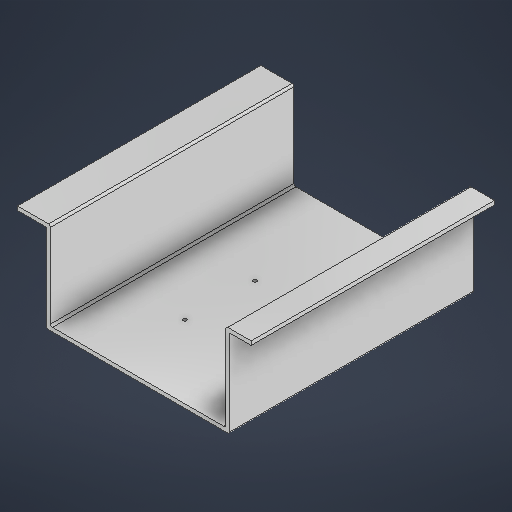
# Autodesk Inventor part: Lower joint housing
Saved by Autodesk Inventor 2026.3 (Build 303398000, 398)
## iProperties
Created: 2026-07-26
Part Number: Lower joint housing
Material: Generic
Document SubType Name: Sheet Metal
Designer: matot
Density: 1 g/cm^3
Sheet Metal Rule: Default_mm
Appearance: Default
Author: matot
Autodesk Inventor part; units mm, degrees
ref_plane "YZ Plane" through (0, 0, 0) normal (1, 0, 0) x (0, 1, 0)
ref_plane "XZ Plane" through (0, 0, 0) normal (0, 1, 0) x (-1, 0, 0)
ref_plane "XY Plane" through (0, 0, 0) normal (0, 0, 1) x (1, 0, 0)
sketch "Sketch1" plane through (0, 0, 0) normal (0, 0, 1) x (1, 0, 0)
  line L0 (98, 0) -> (98, -90)
  line L1 (98, -90) -> (-90, -90)
  line L2 (-90, -90) -> (-90, 0)
  line L3 (120, 4) -> (120, 0)
  line L4 (120, 0) -> (-120, 0)
  line L5 (-120, 0) -> (-120, 4)
  line L6 (-86, 4) -> (94, 4)
  line L7 (94, 4) -> (94, -86)
  line L8 (94, -86) -> (-86, -86)
  line L9 (-86, -86) -> (-86, 4)
  line L10 (-90, 0) -> (-86, 0)
  line L11 (94, 0) -> (98, 0)
  line L12 (-120, 4) -> (-86, 4)
  line L13 (94, 4) -> (120, 4)
  point P0 (0, 0)
  point P1 (0, -4)
  point P2 (120, 2)
  point P3 (98, 0)
  dimension "d0" = 188
  dimension "d1" = 90
  dimension "d3" = 90
  dimension "d4" = 240
  dimension "d5" = 120
  dimension "d8" = 90
  dimension "d9" = 180
  dimension "d10" = 4
  dimension "d13" = 0
  dimension "d14" = 4
  constraints: 28 end point, 8 parallel, 5 horizontal, 5 perpendicular, 2 point on line, 1 midpoint
  measures "d0" distance of L0.end L1.end
  measures "d1" distance of L0.start L0.end
  measures "d3" distance from line of point (0, 0) L2
  measures "d4" distance of L5.end L3.start
  measures "d5" horizontal distance of point (0, -4) point (120, 2)
  measures "d8" distance of L6.end L7.end
  measures "d9" distance of L7.end L8.end
  measures "d10" distance between parallel lines of L0 L7
  measures "d13" distance from line of point (0, 0) L4
  measures "d14" distance between parallel lines of L4 L12
extrude "Extrusion1" add sketch "Sketch1" along normal blind 250 contours L4 L7 L13 L3 | L0 L1 L2 L4 L9 L8 L7 | L4 L5 L12 L9
fillet "Fillet1" radius 2 4 edges at (-86, -86, 125) (-86, 4, 125) (94, 4, 125) (98, -90, 125)
fillet "Fillet2" radius 2 2 edges at (-90, -90, 125) (94, -86, 125)
sketch "Sketch3" plane through (-84, -86, 250) normal (0, 1, 0) x (1, 0, 0)
  line L0 (-2, 0) -> (-2, 250) projected
  line L1 (176, 0) -> (0, 0) projected
  point P0 (84, 250)
  point P1 (114.75, 74.7)
  point P2 (61.25, 74.7)
  dimension "d28" = 53.5
  dimension "d29" = 63.25
  dimension "d30" = 0
  dimension "d31" = 74.7
  measures "d28" distance of point (61.25, 74.7) point (114.75, 74.7)
  measures "d29" distance from line of L0 point (61.25, 74.7)
  measures "d30" vertical distance of point (114.75, 74.7) point (61.25, 74.7)
  measures "d31" distance from line of L1 point (61.25, 74.7)
hole "Hole2" at (30.75, -86, 175.3) at (-22.75, -86, 175.3) direction (0, -1, 0) diameter 3.4587 end through all thread size "M4x0.5" class "6H" standard "ISO Metric profile"
sketch "Sketch4" plane through (-84, -86, 250) normal (0, 1, 0) x (1, 0, 0)
  circle A0 centre (61.25, 74.7) radius 1.7294 projected
  circle A1 centre (114.75, 74.7) radius 1.7294 projected
  point P0 (84, 250)
  point P1 (116.1732, 145.3)
  point P2 (62.6732, 145.3)
  dimension "d39" = 53.5
  dimension "d40" = 70.6
  dimension "d41" = 70.6
  measures "d39" distance of point (62.673, 145.3) point (116.173, 145.3)
  measures "d40" vertical distance of A0.centre point (62.673, 145.3)
  measures "d41" vertical distance of A1.centre point (116.173, 145.3)
hole "Hole3" at (32.1732, -86, 104.7) at (-21.3268, -86, 104.7) direction (0, -1, 0) diameter 3.4587 end through all thread size "M4x0.5" class "6H" standard "ISO Metric profile"
equation "\"BendRadius\" = Thickness"
equation "\"BendReliefWidth\" = Thickness"
equation "\"BendReliefDepth\" = 0.5 * Thickness"
equation "\"CornerReliefSize\" = 4 * Thickness"
equation "\"MinimumRemnant\" = 2 * Thickness"
equation "\"TransitionRadius\" = BendRadius"
equation "\"JacobiRadiusSize\" = BendRadius"
equation "\"GapSize\" = Thickness"
equation "\"Thickness\" = 0.5"
body "Solid1"
